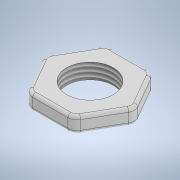
# Autodesk Inventor part: LED Nut
Saved by Autodesk Inventor 2021 (Build 250183000, 183)
## iProperties
Created: 2020-07-20
Part Number: LED Nut
Material: Generic
Document SubType Name: Modeling
Designer: jgray
Density: 1 g/cm^3
Appearance: Default
Author: jgray
Autodesk Inventor part; units mm, degrees
ref_plane "YZ Plane" through (0, 0, 0) normal (1, 0, 0) x (0, 1, 0)
ref_plane "XZ Plane" through (0, 0, 0) normal (0, 1, 0) x (-1, 0, 0)
ref_plane "XY Plane" through (0, 0, 0) normal (0, 0, 1) x (1, 0, 0)
sketch "Sketch1" plane through (0, 0, 0) normal (0, 1, 0) x (-1, 0, 0)
  line L0 (7.0148, -0.75) -> (4.1569, -5.7)
  line L1 (2.8579, -6.45) -> (-2.8579, -6.45)
  line L2 (-4.1569, -5.7) -> (-7.0148, -0.75)
  line L3 (-7.0148, 0.75) -> (-4.1569, 5.7)
  line L4 (-2.8579, 6.45) -> (2.8579, 6.45)
  line L5 (4.1569, 5.7) -> (7.0148, 0.75)
  arc A0 (7.0148, -0.75) -> (7.0148, 0.75) centre (5.7158, 0) ccw
  arc A1 (4.1569, 5.7) -> (2.8579, 6.45) centre (2.8579, 4.95) ccw
  arc A2 (-2.8579, 6.45) -> (-4.1569, 5.7) centre (-2.8579, 4.95) ccw
  arc A3 (-7.0148, 0.75) -> (-7.0148, -0.75) centre (-5.7158, 0) ccw
  arc A4 (-4.1569, -5.7) -> (-2.8579, -6.45) centre (-2.8579, -4.95) ccw
  arc A5 (2.8579, -6.45) -> (4.1569, -5.7) centre (2.8579, -4.95) ccw
  circle A6 centre (0, 0) radius 3.8
  point P0 (7.4478, 0)
  point P1 (3.7239, -6.45)
  point P2 (-3.7239, -6.45)
  point P3 (-7.4478, 0)
  point P4 (-3.7239, 6.45)
  point P5 (3.7239, 6.45)
  dimension "d0" = 12.9
  dimension "d1" = 1.5
  dimension "d2" = 1.5
  dimension "d3" = 7.6
  constraints: 12 end point, 12 point on circle, 12 point on line, 12 tangent, 7 centre point, 4 equal radius, 2 coincident, 13 other
  measures "d0" distance between parallel lines of L3 L0
  measures "d1" radius of A0
  measures "d2" radius of A1
  measures "d3" diameter of A6
extrude "Extrusion1" add sketch "Sketch1" along normal blind 2.5
fillet "Fillet1" radius 0.5 24 edges at (3.6079, 2.5, 6.249) (5.5859, 2.5, 3.225) (7.2158, 2.5, 0) (5.5859, 2.5, -3.225) (3.6079, 2.5, -6.249) (0, 2.5, -6.45) (-3.6079, 2.5, -6.249) (-5.5859, 2.5, -3.225) (-7.2158, 2.5, 0) (-5.5859, 2.5, 3.225) (-3.6079, 2.5, 6.249) (0, 2.5, 6.45) (3.6079, 0, 6.249) (5.5859, 0, 3.225) (7.2158, 0, 0) (5.5859, 0, -3.225) (3.6079, 0, -6.249) (0, 0, -6.45) (-3.6079, 0, -6.249) (-5.5859, 0, -3.225) (-7.2158, 0, 0) (-5.5859, 0, 3.225) (-3.6079, 0, 6.249) (0, 0, 6.45)
thread "Thread1" size "M8x0.75" class "6H" standard "ANSI Metric M Profile" length 12.5
body "Solid1"
